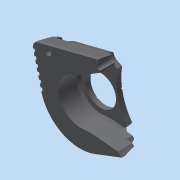
# Autodesk Inventor part: pulleyprotector
Saved by Autodesk Inventor 2014 SP1 (Build 180222100, 222)
## iProperties
Created: 2014-05-23
Part Number: pulleyprotector
Material: Generic
Document SubType Name: Modeling
Designer: brent
Density: 1 g/cm^3
Appearance: Default
d0: 1.000 ul
d1: 0.118 in
d2: 0.236 in
d3: 0.177 in
d5: 0.669 in
d6: 0.00 deg
d31: 1.691 in
d32: 3.543 in
d42: 0.315 in
d43: 0.984 in
d44: 0.157 in
d45: 0.00 deg
d46: 0.100 in
d64: 0.201 in
d65: 0.201 in
d67: 0.00 deg
d68: 0.425 in
d69: 0.425 in
d70: 0.197 in
d71: 0.00 deg
d81: 0.118 in
d82: 0.354 in
d83: 0.00 deg
d98: 0.197 in
d115: 0.591 in
d116: 0.039 in
d117: 150.00 deg
d118: 0.020 in
d119: 0.00 deg
d120: 5.000 ul
d121: 360.00 deg
d125: 0.059 in
d129: 0.00 deg
d130: 0.177 in
d131: 0.100 in
d132: 6.000 ul
d134: 0.200 in
d139: 0.050 in
d140: 0.00 deg
d144: 0.170 in
d148: 0.200 in
d151: 0.200 in
Author: brent
Autodesk Inventor part; units mm, degrees
ref_plane "YZ Plane" through (0, 0, 0) normal (1, 0, 0) x (0, 1, 0)
ref_plane "XZ Plane" through (0, 0, 0) normal (0, 1, 0) x (-1, 0, 0)
ref_plane "XY Plane" through (0, 0, 0) normal (0, 0, 1) x (1, 0, 0)
derived "mount_alt.ipt"
sketch "Sketch22" plane through (-34.72773, 175.742854, 0) normal (0, 0, -1) x (-0.8869066, 0.4619488, 0)
  arc A0 (-24.692007, 66.139919) -> (-35.459367, 72.636875) centre (-47.511586, 40.492002) ccw
  circle A1 centre (0, 0) radius 11
  circle A2 centre (-47.511586, 40.492002) radius 31.83
  circle A3 centre (0, 0) radius 11.935
  line L0 (10.232841, 6.142736) -> (-20.221154, 56.874346)
  line L1 (-59.360681, 10.949695) -> (-4.442945, -11.077205)
  circle A4 centre (0, 0) radius 28
  circle A5 centre (1.296661, 36.642511) radius 2.413
  circle A6 centre (33.935934, 7.602552) radius 2.413
  line L2 (0, 0) -> (-47.511586, 40.492002)
  line L3 (-24.692007, 66.139919) -> (44.692156, 4.407133)
  line L4 (44.901418, 0.821131) -> (24.654276, -21.935512)
  line L5 (-24.654276, -21.935512) -> (-62.459536, 20.555463)
  arc A7 (-24.654276, -21.935512) -> (24.654276, -21.935512) centre (0, 0) ccw
  arc A8 (44.901418, 0.821131) -> (44.692156, 4.407133) centre (43.003786, 2.509501) ccw
  line L6 (-24.692007, 66.139919) -> (44.692156, 4.407133)
  arc A9 (-24.692007, 66.139919) -> (-35.459367, 72.636875) centre (-47.511586, 40.492002) ccw
  arc A10 (-35.459367, 72.636875) -> (-38.463007, 71.669709) centre (-36.351083, 70.258548) ccw
  line L7 (-39.087714, 70.734782) -> (-38.463007, 71.669709)
  arc A11 (-45.202385, 65.893849) -> (-39.087714, 70.734782) centre (-49.647335, 77.790589) ccw
  line L8 (-64.919679, 58.526926) -> (-45.202385, 65.893849)
  arc A12 (-64.919679, 58.526926) -> (-72.37147, 42.185237) centre (-60.47473, 46.630186) ccw
  line L9 (-67.276695, 28.549262) -> (-72.37147, 42.185237)
  arc A13 (-67.276695, 28.549262) -> (-62.459536, 20.555463) centre (-43.483214, 37.43916) ccw
  line L10 (-24.654276, -21.935512) -> (-62.459536, 20.555463)
  arc A14 (-24.654276, -21.935512) -> (24.654276, -21.935512) centre (0, 0) ccw
  line L11 (44.901418, 0.821131) -> (24.654276, -21.935512)
  ellipse E0 centre (-42.955135, 42.194417) end of major axis (-46.111049, 50.641103) minor radius 5.207074 (-39.799221, 33.747732) -> (-38.060609, 43.971716) ccw
  line L12 (-39.799221, 33.747732) -> (-51.487768, 29.380569)
  arc A15 (-54.551835, 30.77778) -> (-51.487768, 29.380569) centre (-52.321196, 31.611208) ccw
  line L13 (-54.551835, 30.77778) -> (-59.641302, 44.399548)
  arc A16 (-58.244091, 47.463614) -> (-59.641302, 44.399548) centre (-57.410663, 45.232975) ccw
  line L14 (-58.244091, 47.463614) -> (-43.908519, 52.819778)
  arc A17 (-40.844452, 51.422567) -> (-43.908519, 52.819778) centre (-43.075091, 50.589139) ccw
  line L15 (-40.844452, 51.422567) -> (-38.060609, 43.971716)
  circle A18 centre (0, 0) radius 11
  circle A19 centre (-21.198971, 10.929654) radius 2.15
  circle A20 centre (-16.87996, -13.401891) radius 2.15
  circle A21 centre (13.616103, -19.565507) radius 2.15
  circle A22 centre (19.779719, 10.930556) radius 2.15
  circle A23 centre (-10.716344, 17.094172) radius 2.15
  circle A24 centre (-11.143867, -18.513424) radius 2.15
  circle A25 centre (18.299212, -8.458319) radius 2.15
  circle A26 centre (8.244107, 20.984759) radius 2.15
  circle A27 centre (-1.749269, 21.930346) radius 2.15
  circle A28 centre (-21.930346, -1.749269) radius 2.15
  circle A29 centre (1.749269, -21.930346) radius 2.15
  circle A30 centre (21.930346, 1.749269) radius 2.15
  point P0 (-111.984448, -139.825066)
sketch "Sketch2" plane through (0, 0, 0) normal (0, 0, 1) x (1, 0, 0)
  circle A0 centre (-61.313745, 198.16227) radius 2.413
  circle A1 centre (-18.950785, 208.84033) radius 2.413
  circle A2 centre (-34.72773, 175.742854) radius 11.935
  line L0 (22.977848, 158.032618) -> (-35.904354, 163.865994)
  line L1 (-40.965675, 185.917934) -> (9.479578, 216.84395)
  circle A3 centre (26.11584, 189.707559) radius 31.83
  circle A4 centre (-34.72773, 175.742854) radius 28
  arc A5 (-7.887117, 160.232164) -> (-17.337126, 201.405411) centre (-34.72773, 175.742854) ccw
  arc A6 (-29.202788, 158.680051) -> (-37.196243, 193.507162) centre (-34.72773, 175.742854) ccw
  line L2 (-37.196243, 193.507162) -> (-23.991249, 201.602629)
  arc A7 (-0.530038, 153.444669) -> (-10.4864, 215.885336) centre (26.11584, 189.707559) ccw
  line L3 (-28.195318, 145.438933) -> (-59.424621, 138.707042)
  line L4 (-20.908765, 203.492379) -> (-18.921093, 204.710943)
  line L5 (-4.646578, 213.462091) -> (-5.569762, 217.12463)
  line L6 (-74.171774, 197.213275) -> (-66.726853, 167.677115)
  line L7 (17.725028, 222.996343) -> (-72.329629, 200.297055)
  line L8 (-74.171774, 197.213275) -> (-74.792592, 199.676238)
  line L9 (-72.329629, 200.297055) -> (-74.792592, 199.676238)
  line L10 (-66.726853, 167.677115) -> (-59.424621, 138.707042)
  arc A8 (-66.726853, 167.677115) -> (-22.994773, 144.899091) centre (-34.72773, 175.742854) ccw
  line L11 (-22.994773, 144.899091) -> (30.163615, 165.120524)
  arc A9 (-7.887117, 160.232164) -> (-6.479635, 158.68281) centre (26.11584, 189.707559) ccw
  arc A10 (-17.337126, 201.405411) -> (-17.639427, 200.218347) centre (26.11584, 189.707559) ccw
  arc A11 (-10.4864, 215.885336) -> (-15.511033, 206.801518) centre (26.11584, 189.707559) ccw
  arc A12 (-8.6768, 161.168599) -> (-7.887117, 160.232164) centre (26.11584, 189.707559) ccw
  arc A13 (-10.191235, 156.796603) -> (-7.887117, 160.232164) centre (-34.72773, 175.742854) ccw
  arc A14 (-17.337126, 201.405411) -> (-10.191235, 156.796603) centre (-34.72773, 175.742854) ccw
  arc A15 (-17.639427, 200.218347) -> (-18.066613, 198.246346) centre (26.11584, 189.707559) ccw
  arc A16 (-18.066613, 198.246346) -> (-18.408592, 183.182607) centre (26.11584, 189.707559) ccw
  arc A17 (-15.511033, 206.801518) -> (-17.337126, 201.405411) centre (26.11584, 189.707559) ccw
  line L12 (-29.202788, 158.680051) -> (-13.789264, 157.153055)
  arc A18 (-9.921152, 162.756951) -> (-8.6768, 161.168599) centre (26.11584, 189.707559) ccw
  arc A19 (-18.408592, 183.182607) -> (-9.921152, 162.756951) centre (26.11584, 189.707559) ccw
  line L13 (-13.789264, 157.153055) -> (-10.191235, 156.796603)
  line L14 (-10.191235, 156.796603) -> (-3.890735, 156.172421)
  line L15 (-23.991249, 201.602629) -> (-20.908765, 203.492379)
  line L16 (-15.511033, 206.801518) -> (-4.646578, 213.462091)
  line L17 (-18.921093, 204.710943) -> (-15.511033, 206.801518)
  arc A20 (-37.196243, 193.507162) -> (-29.202788, 158.680051) centre (-34.72773, 175.742854) ccw
  arc A21 (-3.890735, 156.172421) -> (-0.530038, 153.444669) centre (26.11584, 189.707559) ccw
  arc A22 (-6.479635, 158.68281) -> (-3.890735, 156.172421) centre (26.11584, 189.707559) ccw
  point P0 (0, 0)
  point P1 (-29.756676, 166.607909)
  point P2 (-35.904354, 163.865994)
  point P3 (-34.329229, 188.394009)
  point P4 (9.479578, 216.84395)
  dimension "d1" = 3
  dimension "d2" = 6
  dimension "d3" = 4.5
  dimension "d32" = 90
  dimension "d115" = 15
  dimension "d130" = 4.5
  constraints: 46 point on circle, 26 end point, 17 centre point, 6 collinear, 4 perpendicular, 3 coincident, 3 point on line, 3 tangent, 10 other
  measures "d1" radial gap between concentric circles of A5 A4
  measures "d32" diameter of A7
  measures "d115" distance from line of A1.centre L5
extrude "Extrusion1" add sketch "Sketch2" along normal blind 17 contours A20 L12 A4 L2 | A4 L13 A14 L15 | A14 L3 A8 L6 L8 L9 L7 A11 L17 L4 | L14 A21 L11 A8 L3 A14
fillet "Fillet3" radius 42.9625 2 edges at (-37.1962, 193.5072, 8.5) (-29.2028, 158.6801, 8.5)
sketch "Sketch6" plane through (0, 0, 0) normal (0, 0, -1) x (-1, 0, 0)
  arc A0 (32.515453, 157.944818) -> (40.49797, 192.724272) centre (34.72773, 175.742854) ccw
  circle A1 centre (34.72773, 175.742854) radius 25.935
  circle A2 centre (34.72773, 175.742854) radius 12.5
  point P0 (0, 0)
  dimension "d42" = 8
  dimension "d43" = 25
  constraints: 2 centre point, 2 coincident
  measures "d42" radial gap between concentric circles of A1 A0
  measures "d43" diameter of A2
extrude "Extrusion7" add sketch "Sketch6" along normal blind 4
chamfer "Chamfer6" distance 2.54 angle 45 2 edges at (-49.7577, 196.8787, 0) (-44.6487, 151.7804, 0)
chamfer "Chamfer14" distance 1.5 angle 45 3 edges at (-36.069, 194.5095, 0) (-29.0394, 198.5078, 0) (-27.7513, 158.2696, 0)
sketch "Sketch9" plane through (0, 0, 0) normal (0, 0, -1) x (-1, 0, 0)
  circle A0 centre (61.313745, 198.16227) radius 2.5527
  circle A1 centre (18.950785, 208.84033) radius 2.5527
  point P0 (0, 0)
  dimension "d64" = 5.1054
  dimension "d65" = 5.1054
  constraints: 2 centre point, 2 coincident
  measures "d64" diameter of A0
  measures "d65" diameter of A1
extrude "Extrusion9" cut sketch "Sketch9" against normal through all
sketch "Sketch10" plane through (0, 0, 0) normal (0, 0, -1) x (-1, 0, 0)
  arc A0 (63.866445, 198.16227) -> (63.866445, 198.16227) centre (61.313745, 198.16227) ccw
  circle A1 centre (18.950785, 208.84033) radius 2.5527
  circle A2 centre (18.950785, 208.84033) radius 5.3975
  circle A3 centre (61.313745, 198.16227) radius 5.3975
  point P0 (0, 0)
  dimension "d68" = 10.795
  dimension "d69" = 10.795
  constraints: 2 centre point, 2 coincident
  measures "d68" diameter of A2
  measures "d69" diameter of A3
extrude "Extrusion10" cut sketch "Sketch10" against normal blind 5 contours A0 | A2 | A3
sketch "Sketch12" plane through (0, 0, -4) normal (0, 0, -1) x (-1, 0, 0)
  circle A0 centre (-26.11584, 189.707559) radius 45
  circle A1 centre (-26.11584, 189.707559) radius 48
  point P0 (0, 0)
  dimension "d81" = 3
  constraints: 1 centre point, 1 coincident
  measures "d81" radial gap between concentric circles of A0 A1
extrude "Extrusion12" cut sketch "Sketch12" against normal blind 9 contours A0 | A1
fillet "Fillet10" radius 5 1 edges at (-74.7926, 199.6762, 8.5)
sketch "Sketch14" plane through (0, 0, 5) normal (0, 0, -1) x (-1, 0, 0)
  line L0 (20.579295, 203.694364) -> (15.511033, 206.801518)
  arc A0 (20.579295, 203.694364) -> (22.577781, 212.837568) centre (18.950785, 208.84033) ccw
  circle A1 centre (18.950785, 208.84033) radius 2.5527
  line L1 (18.168419, 205.172378) -> (19.942113, 213.487957)
  line L2 (20.579295, 203.694364) -> (15.511033, 206.801518)
  line L3 (60.014815, 203.401143) -> (64.940741, 202.159508)
  arc A2 (3.825836, 152.190948) -> (8.683831, 156.647267) centre (-26.11584, 189.707559) ccw
  line L4 (19.942113, 213.487957) -> (3.615842, 221.213261)
  line L5 (3.615842, 221.213261) -> (-2.764215, 200.830659)
  line L6 (18.168419, 205.172378) -> (-2.764215, 200.830659)
  arc A3 (15.511033, 206.801518) -> (10.4864, 215.885336) centre (-26.11584, 189.707559) ccw
  line L7 (10.4864, 215.885336) -> (14.805226, 214.796727)
  arc A4 (60.014815, 203.401143) -> (64.940741, 202.159508) centre (61.313745, 198.16227) ccw
  line L8 (3.890735, 156.172421) -> (8.683831, 156.647267)
  arc A5 (0.530038, 153.444669) -> (3.890735, 156.172421) centre (-26.11584, 189.707559) ccw
  line L9 (3.825836, 152.190948) -> (0.530038, 153.444669)
  arc A6 (17.651855, 214.079203) -> (15.749977, 213.186344) centre (18.950785, 208.84033) ccw
  line L10 (17.651855, 214.079203) -> (22.577781, 212.837568)
  arc A7 (15.749977, 213.186344) -> (14.805226, 214.796727) centre (-26.11584, 189.707559) ccw
  point P0 (0, 0)
  point P1 (4.646578, 213.462091)
  point P2 (20.051305, 202.845091)
  constraints: 8 end point, 1 point on line, 2 other
extrude "Extrusion17" cut sketch "Sketch14" along normal through all both and the other way through all contours L6 L5 L4 L10 A6 A7 L7 A3 L0 | L0 A3 L7 A7 A6 L10 L4 L1 A1 | L1 A1 | A1 L1
chamfer "Chamfer16" distance 4.318 angle 45 6 edges at (-70.1487, 181.2525, 0) (-49.972, 146.4749, 0) (-13.4103, 148.545, 0) (-73.0146, 198.6141, 0) (-67.4425, 201.5289, 0) (-41.2963, 208.1194, 0)
chamfer "Chamfer17" distance 5.08 angle 45 5 edges at (-70.1487, 181.2525, 4.318) (-73.0146, 198.6141, 4.318) (-67.4425, 201.5289, 4.318) (-49.972, 146.4749, 4.318) (-13.4103, 148.545, 4.318)
chamfer "Chamfer18" distance 5.08 angle 45 5 edges at (-49.972, 146.4749, 9.398) (-70.1487, 181.2525, 9.398) (-73.0146, 198.6141, 9.398) (-44.9116, 207.2081, 9.398) (-11.7624, 149.1719, 9.398)
sketch "Sketch18" plane through (-66.726853, 167.677115, 0) normal (-0.9696704, -0.2444163, 0) x (0, 0, 1)
  line L0 (17, 28) -> (17, 0) projected
  line L1 (0, 28) -> (17, 28)
  line L2 (17, 28) -> (17, 25.46)
  line L3 (17, 25.46) -> (0, 25.46)
  line L4 (0, 25.46) -> (0, 28)
  line L5 (0, 22.92) -> (17, 22.92)
  line L6 (17, 22.92) -> (17, 20.38)
  line L7 (17, 20.38) -> (0, 20.38)
  line L8 (0, 20.38) -> (0, 22.92)
  line L9 (0, 17.84) -> (17, 17.84)
  line L10 (17, 17.84) -> (17, 15.3)
  line L11 (17, 15.3) -> (0, 15.3)
  line L12 (0, 15.3) -> (0, 17.84)
  line L13 (0, 12.76) -> (17, 12.76)
  line L14 (17, 12.76) -> (17, 10.22)
  line L15 (17, 10.22) -> (0, 10.22)
  line L16 (0, 10.22) -> (0, 12.76)
  line L17 (0, 7.68) -> (17, 7.68)
  line L18 (17, 7.68) -> (17, 5.14)
  line L19 (17, 5.14) -> (0, 5.14)
  line L20 (0, 5.14) -> (0, 7.68)
  line L21 (0, 2.6) -> (17, 2.6)
  line L22 (17, 2.6) -> (17, 0.06)
  line L23 (17, 0.06) -> (0, 0.06)
  line L24 (0, 0.06) -> (0, 2.6)
  point P0 (0, -178.900665)
  dimension "d131" = 2.54
  dimension "d134" = 5.08
  constraints: 48 end point, 2 parallel, 1 horizontal, 1 perpendicular, 1 point on line, 1 vertical, 40 other
  measures "d131" distance between parallel lines of L1 L3
  measures "d134" distance of L1.start L5.start
extrude "Extrusion18" cut sketch "Sketch18" against normal blind 1.27
sketch "Sketch16" plane through (0, 0, -4) normal (0, 0, -1) x (-1, 0, 0)
  circle A0 centre (34.72773, 175.742854) radius 12.5
  arc A1 (12.896315, 161.74237) -> (21.186431, 197.862018) centre (-26.11584, 189.707559) ccw
  arc A2 (12.896315, 161.74237) -> (21.186431, 197.862018) centre (34.72773, 175.742854) ccw
  line L0 (34.72773, 175.742854) -> (34.72773, 188.242854)
  line L1 (34.72773, 188.242854) -> (41.900398, 200.666278)
  line L2 (35.853123, 188.19209) -> (42.88013, 200.363223)
  arc A3 (41.900398, 200.666278) -> (21.186431, 197.862018) centre (34.72773, 175.742854) ccw
  arc A4 (42.88013, 200.363223) -> (41.900398, 200.666278) centre (34.72773, 175.742854) ccw
  arc A5 (35.853123, 188.19209) -> (34.72773, 188.242854) centre (34.72773, 175.742854) ccw
  arc A6 (34.72773, 188.242854) -> (35.853123, 188.19209) centre (34.72773, 175.742854) ccw
  point P0 (0, 0)
  dimension "d116" = 1
  dimension "d117" = 150
  constraints: 11 point on circle, 6 end point, 4 centre point, 2 coincident, 1 parallel, 1 vertical
  measures "d116" distance between parallel lines of L1 L2
  measures "d117" angle of L1 L0
extrude "Extrusion15" cut sketch "Sketch16" against normal blind 0.5 contours A0 L1 A2 L2
pattern_circular "Circular Pattern1" count 5 over 360 about axis through (-34.72773, 175.742854, 0) along (0, 0, -1) of "Extrusion15"
body "Solid1"
